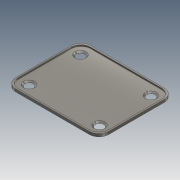
# Autodesk Inventor part: capa de alguma parte da guitarra
Saved by Autodesk Inventor 2016 (Build 200138000, 138)
## iProperties
Created: 2018-10-31
Part Number: capa de alguma parte da guitarra
Material: Genérico
Document SubType Name: Modeling
Designer: thiag
Density: 1 g/cm^3
Appearance: Steel - Polished
Author: thiag
Autodesk Inventor part; units mm, degrees
ref_plane "YZ Plane" through (0, 0, 0) normal (1, 0, 0) x (0, 1, 0)
ref_plane "XZ Plane" through (0, 0, 0) normal (0, 1, 0) x (-1, 0, 0)
ref_plane "XY Plane" through (0, 0, 0) normal (0, 0, 1) x (1, 0, 0)
sketch "Esboço1" plane through (0, 0, 0) normal (0, 0, 1) x (1, 0, 0)
  line L0 (-14.4362, 6.271) -> (52.5638, 6.271)
  line L1 (52.5638, 6.271) -> (52.5638, -47.729)
  line L2 (52.5638, -47.729) -> (-14.4362, -47.729)
  line L3 (-14.4362, -47.729) -> (-14.4362, 6.271)
  circle A0 centre (-6.2862, -2.229) radius 3
  circle A1 centre (-6.2862, -39.229) radius 3
  circle A2 centre (44.4138, -39.229) radius 3
  circle A3 centre (44.4138, -2.229) radius 3
  point P0 (0, 0)
  dimension "d0" = 67
  dimension "d1" = 54
  dimension "d6" = 6
  dimension "d7" = 6
  dimension "d8" = 6
  dimension "d9" = 6
  dimension "d17" = 50.7
  dimension "d18" = 50.7
  dimension "d19" = 37
  dimension "d20" = 37
  dimension "d21" = 8.15
  dimension "d22" = 8.5
  dimension "d24" = 8.15
  dimension "d26" = 8.5
  dimension "d27" = 8.15
  dimension "d28" = 8.15
  dimension "d29" = 8.5
  dimension "d30" = 8.5
  constraints: 8 end point, 4 centre point, 2 parallel, 1 horizontal, 1 perpendicular
  measures "d0" distance of L1.end L2.end
  measures "d1" distance of L0.end L1.end
  measures "d6" diameter of A0
  measures "d7" diameter of A1
  measures "d8" diameter of A2
  measures "d9" diameter of A3
  measures "d17" distance of A3.centre A0.centre
  measures "d18" distance of A2.centre A1.centre
  measures "d19" distance of A1.centre A0.centre
  measures "d20" distance of A2.centre A3.centre
  measures "d21" distance from line of L3 A0.centre
  measures "d22" distance from line of L0 A0.centre
  measures "d24" distance from line of L1 A3.centre
  measures "d26" distance from line of L2 A2.centre
  measures "d27" distance from line of L3 A1.centre
  measures "d28" distance from line of L1 A2.centre
  measures "d29" distance from line of L0 A3.centre
  measures "d30" distance from line of L2 A1.centre
extrude "Extrusão1" add sketch "Esboço1" along normal blind 2
shell "Casca1" thickness 1 removed faces 5 at (11.3623, -15.2254, 2) at (-3.2959, -39.4704, 1.3333) at (-3.2959, -2.4704, 1.3333) at (47.4041, -2.4704, 1.3333) at (47.4041, -39.4704, 1.3333)
chamfer "Chanfro1" distance 1 angle 45 4 edges at (-9.2862, -39.229, 1) (-9.2862, -2.229, 1) (41.4138, -2.229, 1) (41.4138, -39.229, 1)
fillet "Arredondamento1" radius 7 8 edges at (-13.4362, 5.271, 1.5) (-14.4362, 6.271, 1) (52.5638, 6.271, 1) (51.5638, 5.271, 1.5) (51.5638, -46.729, 1.5) (52.5638, -47.729, 1) (-13.4362, -46.729, 1.5) (-14.4362, -47.729, 1)
